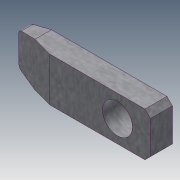
# Autodesk Inventor part: J005776
Saved by Autodesk Inventor 2015 SP1 (Build 190203100, 203)
## iProperties
Created: 2007-05-23
Part Number: J005776
Document SubType Name: Modeling
Designer: komiyamat
Density: 8 g/cm^3
Material: STAINLESS STEEL, 303
Description: HEAD POST HOLDER TOP
Appearance: Metal-Steel (Stainless, Brushed)
Project: COMMON
Vendor: HHMI: JRC - ID&F
ALTERED ITEM DESCRIPTION: N/A
ALTERED ITEM PART NUMBER: N/A
ALTERED ITEM VENDOR: N/A
SPECIAL FINISH: NONE
SURFACE ROUGHNESS: 63 Ra
DESIGN DEPARTMENT: HHMI: JRC - ID&F
LAB/DEPT: COMMON
REQUESTING SCIENTIST: COMMON
Author: komiyamat
Revision Number: -
Autodesk Inventor part; units mm, degrees
ref_plane "YZ Plane" through (0, 0, 0) normal (1, 0, 0) x (0, 1, 0)
ref_plane "XZ Plane" through (0, 0, 0) normal (0, 1, 0) x (-1, 0, 0)
ref_plane "XY Plane" through (0, 0, 0) normal (0, 0, 1) x (1, 0, 0)
sketch "Sketch1" plane through (0, 0, 0) normal (0, 0, 1) x (1, 0, 0)
  line L0 (-25.4, 6.35) -> (-25.4, 0)
  line L1 (-25.4, 0) -> (-4.7625, 0)
  line L2 (-4.7625, 0) -> (-4.7625, 6.35)
  line L3 (-4.7625, 6.35) -> (-25.4, 6.35)
  dimension "d0" = 6.35
  dimension "d1" = 20.6375
  constraints: 8 end point, 2 parallel, 1 perpendicular, 1 vertical
  measures "d0" distance of L0.start L0.end
  measures "d1" distance of L0.end L1.end
extrude "Extrusion1" add sketch "Sketch1" along normal blind 3.175
hole "Hole1" at (-9.525, 3.175, 3.175) direction (0, 0, -1) diameter 4.318 end through all clearance for "Flat Head Machine Screw (82)" size "#8" standard "Ansi Unified Screw Threads"
chamfer "Chamfer3" distance 0.7937 angle 45 1 edges at (-4.7625, 0, 1.5875)
chamfer "Chamfer4" distance 0.7937 angle 45 1 edges at (-4.7625, 6.35, 1.5875)
chamfer "Chamfer5" distance 0.7937 distance2 3.175 1 edges at (-25.4, 0, 1.5875) measured on face at (-25.4, 4.2333, 1.0583)
chamfer "Chamfer6" distance 3.175 distance2 0.7937 1 edges at (-25.4, 6.35, 1.5875) measured on face at (-12.1708, 6.35, 1.0583)
chamfer "Chamfer7" distance 6.096 angle 15 1 edges at (-25.4, 3.175, 3.175) measured on face at (-18.7061, 3.2617, 3.175)
fillet "Fillet1" radius 0.635 2 edges at (-25.4, 0.7937, 0.7708) (-25.4, 5.5562, 0.7708)
body "Solid1"
